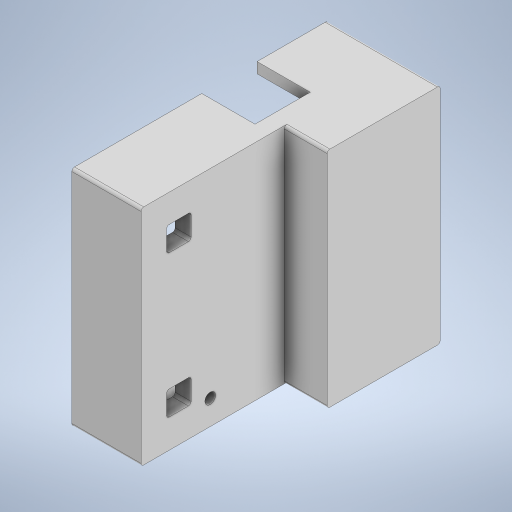
# Autodesk Inventor part: Part1
Saved by Autodesk Inventor 2023 (Build 270158030, 158C)
## iProperties
Created: 2023-07-27
Part Number: Part1
Material: Generic
Document SubType Name: Modeling
Designer: Tropaion
Density: 1 g/cm^3
Appearance: Default
Author: Tropaion
Autodesk Inventor part; units mm, degrees
ref_plane "YZ Plane" through (0, 0, 0) normal (1, 0, 0) x (0, 1, 0)
ref_plane "XZ Plane" through (0, 0, 0) normal (0, 1, 0) x (-1, 0, 0)
ref_plane "XY Plane" through (0, 0, 0) normal (0, 0, 1) x (1, 0, 0)
sketch "Sketch2" plane through (0, 0, 0) normal (1, 0, 0) x (0, 1, 0)
  line L0 (5.574, -18.3788) -> (-36.426, -18.3788)
  line L1 (-36.426, -18.3788) -> (-36.426, -39.5888)
  line L2 (-36.426, -39.5888) -> (5.574, -39.5888)
  line L3 (5.574, -39.5888) -> (5.574, -18.3788)
  point P0 (0, 0)
  dimension "d0" = 42
  dimension "d1" = 21.21
  constraints: 8 end point, 2 parallel, 1 horizontal, 1 perpendicular
  measures "d0" distance of L2.end L1.end
  measures "d1" distance of L1.end L0.end
extrude "Extrusion1" add sketch "Sketch2" along normal blind 3
sketch "Sketch4" plane through (0, 0, 0) normal (-1, 0, 0) x (0, 0, 1)
  line L0 (-18.3788, -36.426) -> (-39.5888, -36.426) projected
  line L1 (-39.5888, 5.574) -> (-18.3788, 5.574) projected
  line L2 (-18.3788, -36.426) -> (-21.3788, -36.426)
  line L3 (-21.3788, -36.426) -> (-21.3788, 5.574)
  line L4 (-21.3788, 5.574) -> (-18.3788, 5.574)
  line L5 (-18.3788, 5.574) -> (-18.3788, -36.426)
  point P0 (0, 0)
  point P1 (-18.3788, 5.574)
  dimension "d5" = 3
  constraints: 8 end point, 2 parallel, 1 horizontal, 1 perpendicular, 1 point on line
  measures "d5" distance of L3.end L4.end
extrude "Extrusion2" add sketch "Sketch4" along normal blind 8.09
sketch "Sketch5" plane through (3, -36.426, -18.3788) normal (0, 0, 1) x (1, 0, 0)
  line L0 (0, 0) -> (-11.09, 0) projected
  line L1 (-11.09, 42) -> (0, 42) projected
  line L2 (-11.09, 0) -> (-8.09, 0)
  line L3 (-8.09, 0) -> (-8.09, 42)
  line L4 (-8.09, 42) -> (-11.09, 42)
  line L5 (-11.09, 42) -> (-11.09, 0)
  point P0 (-3, 36.426)
  dimension "d8" = 3
  constraints: 8 end point, 2 parallel, 1 horizontal, 1 perpendicular, 1 point on line
  measures "d8" distance of L4.end L3.end
extrude "Extrusion3" add sketch "Sketch5" along normal blind 26.9
sketch "Sketch6" plane through (-8.09, 0, 0) normal (-1, 0, 0) x (0, 0, 1)
  line L0 (8.5212, 5.574) -> (8.5212, -36.426) projected
  line L1 (-21.3788, 5.574) -> (8.5212, 5.574)
  line L2 (8.5212, 5.574) -> (8.5212, 3.574)
  line L3 (8.5212, 3.574) -> (-21.3788, 3.574)
  line L4 (-21.3788, 3.574) -> (-21.3788, 5.574)
  point P0 (0, 0)
  dimension "d11" = 2
  constraints: 8 end point, 2 parallel, 1 horizontal, 1 perpendicular, 1 point on line
  measures "d11" distance of L1.end L2.end
extrude "Extrusion4" add sketch "Sketch6" along normal blind 10
sketch "Sketch7" plane through (0, 0, 0) normal (-1, 0, 0) x (0, 0, 1)
  line L0 (-21.3788, -36.426) -> (-21.3788, 5.574) projected
  line L1 (-39.5888, 5.574) -> (-21.3788, 5.574)
  line L2 (-21.3788, 5.574) -> (-21.3788, 3.574)
  line L3 (-21.3788, 3.574) -> (-39.5888, 3.574)
  line L4 (-39.5888, 3.574) -> (-39.5888, 5.574)
  point P0 (0, 0)
  dimension "d14" = 2
  constraints: 8 end point, 2 parallel, 1 horizontal, 1 perpendicular, 1 point on line
  measures "d14" distance of L1.end L2.end
extrude "Extrusion5" add sketch "Sketch7" along normal blind 18.09
sketch "Sketch8" plane through (-8.09, 0, 0) normal (-1, 0, 0) x (0, 0, 1)
  line L0 (-18.3788, -36.426) -> (8.5212, -36.426) projected
  line L1 (-21.3788, -36.426) -> (-21.3788, 3.574) projected
  line L2 (8.5212, -36.426) -> (-21.3788, -36.426)
  line L3 (-21.3788, -36.426) -> (-21.3788, -34.026)
  line L4 (-21.3788, -34.026) -> (8.5212, -34.026)
  line L5 (8.5212, -34.026) -> (8.5212, -36.426)
  point P0 (0, 0)
  dimension "d17" = 2.4
  constraints: 8 end point, 2 parallel, 1 horizontal, 1 perpendicular, 1 point on line
  measures "d17" distance of L2.end L3.end
extrude "Extrusion6" add sketch "Sketch8" along normal blind 10
sketch "Sketch9" plane through (0, 0, 0) normal (-1, 0, 0) x (0, 0, 1)
  line L0 (-39.5888, -36.426) -> (-39.5888, 5.574) projected
  line L1 (-21.3788, 3.574) -> (-21.3788, -34.026) projected
  line L2 (-39.5888, -36.426) -> (-21.3788, -36.426)
  line L3 (-21.3788, -36.426) -> (-21.3788, -34.026)
  line L4 (-21.3788, -34.026) -> (-39.5888, -34.026)
  line L5 (-39.5888, -34.026) -> (-39.5888, -36.426)
  point P0 (0, 0)
  constraints: 8 end point, 2 parallel, 1 horizontal, 1 perpendicular
extrude "Extrusion7" add sketch "Sketch9" along normal blind 18.09
sketch "Sketch10" plane through (-8.09, 0, 0) normal (-1, 0, 0) x (0, 0, 1)
  line L0 (-39.5888, 3.574) -> (8.5212, 3.574) projected
  line L1 (8.5212, -34.026) -> (-39.5888, -34.026) projected
  line L2 (8.5212, 3.574) -> (6.1212, 3.574)
  line L3 (6.1212, 3.574) -> (6.1212, -34.026)
  line L4 (6.1212, -34.026) -> (8.5212, -34.026)
  line L5 (8.5212, -34.026) -> (8.5212, 3.574)
  point P0 (0, 0)
  dimension "d22" = 2.4
  constraints: 8 end point, 2 parallel, 1 horizontal, 1 perpendicular, 1 point on line
  measures "d22" distance of L4.end L3.end
extrude "Extrusion8" add sketch "Sketch10" along normal blind 10
sketch "Sketch11" plane through (0, 0, 0) normal (-1, 0, 0) x (0, 0, 1)
  line L0 (-39.5888, 3.574) -> (6.1212, 3.574) projected
  line L1 (6.1212, -34.026) -> (-39.5888, -34.026) projected
  line L2 (-39.5888, 3.574) -> (-37.1888, 3.574)
  line L3 (-37.1888, 3.574) -> (-37.1888, -34.026)
  line L4 (-37.1888, -34.026) -> (-39.5888, -34.026)
  line L5 (-39.5888, -34.026) -> (-39.5888, 3.574)
  point P0 (0, 0)
  dimension "d25" = 2.4
  constraints: 8 end point, 2 parallel, 1 horizontal, 1 perpendicular, 1 point on line
  measures "d25" distance of L3.end L4.end
extrude "Extrusion9" add sketch "Sketch11" along normal blind 18.09
sketch "Sketch13" plane through (3, -36.426, -39.5888) normal (0, 0, -1) x (-1, 0, 0)
  line L0 (21.09, 40) -> (21.09, 2.4) projected
  line L1 (21.09, 3.2) -> (3.09, 3.2)
  line L2 (3.09, 3.2) -> (3.09, 16.4)
  line L3 (3.09, 16.4) -> (21.09, 16.4)
  line L4 (21.09, 16.4) -> (21.09, 3.2)
  line L5 (21.09, 0) -> (0, 0) projected
  point P0 (3, 36.426)
  dimension "d28" = 18
  dimension "d29" = 13.2
  dimension "d30" = 3.2
  constraints: 8 end point, 2 parallel, 1 horizontal, 1 perpendicular, 1 point on line
  measures "d28" distance of L2.end L3.end
  measures "d29" distance of L1.end L2.end
  measures "d30" distance between parallel lines of L5 L1
extrude "RJ12" cut sketch "Sketch13" against normal blind 2.4
sketch "Sketch14" plane through (3, -36.426, -39.5888) normal (0, 0, -1) x (-1, 0, 0)
  line L0 (21.09, 0) -> (21.09, 42) projected
  line L1 (21.09, 39.5) -> (5.89, 39.5)
  line L2 (5.89, 39.5) -> (5.89, 25.6)
  line L3 (5.89, 25.6) -> (21.09, 25.6)
  line L4 (21.09, 25.6) -> (21.09, 39.5)
  line L5 (21.09, 42) -> (0, 42) projected
  point P0 (3, 36.426)
  point P1 (21.09, 25.6)
  dimension "d33" = 15.2
  dimension "d34" = 13.9
  dimension "d35" = 2.5
  constraints: 8 end point, 2 parallel, 1 horizontal, 1 perpendicular, 1 point on line
  measures "d33" distance of L3.end L2.end
  measures "d34" distance of L2.end L1.end
  measures "d35" distance between parallel lines of L5 L1
extrude "PowerConnector" cut sketch "Sketch14" against normal blind 2.4
sketch "Sketch15" plane through (3, -36.426, -39.5888) normal (0, 0, -1) x (-1, 0, 0)
  line L0 (5.89, 39.5) -> (5.89, 25.6) projected
  line L1 (5.89, 33.6) -> (3.39, 33.6)
  line L2 (3.39, 33.6) -> (3.39, 31.6)
  line L3 (3.39, 31.6) -> (5.89, 31.6)
  line L4 (5.89, 31.6) -> (5.89, 33.6)
  line L5 (5.89, 39.5) -> (21.09, 39.5) projected
  point P0 (3, 36.426)
  point P1 (4.64, 33.6)
  dimension "d38" = 2.5
  dimension "d39" = 2
  dimension "d40" = 5.9
  constraints: 8 end point, 2 parallel, 1 horizontal, 1 midpoint, 1 perpendicular, 1 point on line
  measures "d38" distance of L3.end L2.end
  measures "d39" distance of L2.end L1.end
  measures "d40" distance from line of point (4.64, 33.6) L5
extrude "PowerConnector2" cut sketch "Sketch15" against normal blind 2.4
sketch "Sketch16" plane through (3, 5.574, -18.3788) normal (0, 1, 0) x (1, 0, 0)
  line L0 (-21.09, 18.81) -> (-21.09, -24.5) projected
  line L1 (-21.09, 7.91) -> (-11.09, 7.91)
  line L2 (-11.09, 7.91) -> (-11.09, -2.49)
  line L3 (-11.09, -2.49) -> (-21.09, -2.49)
  line L4 (-21.09, -2.49) -> (-21.09, 7.91)
  line L5 (-21.09, 21.21) -> (0, 21.21) projected
  point P0 (-3, -18.3788)
  dimension "d43" = 10
  dimension "d44" = 10.4
  dimension "d45" = 13.3
  constraints: 8 end point, 2 parallel, 1 horizontal, 1 perpendicular, 1 point on line
  measures "d43" distance of L2.end L3.end
  measures "d44" distance of L1.end L2.end
  measures "d45" distance between parallel lines of L5 L1
extrude "USBC" cut sketch "Sketch16" against normal blind 2.4
sketch "Sketch17" plane through (-5.09, -36.426, -18.3788) normal (1, 0, 0) x (0, 0, -1)
  line L0 (-17.5, 36.75) -> (-22.1, 36.75)
  line L1 (-22.1, 36.75) -> (-22.1, 32.15)
  line L2 (-22.1, 32.15) -> (-17.5, 32.15)
  line L3 (-17.5, 32.15) -> (-17.5, 36.75)
  line L4 (0, 42) -> (-26.9, 42) projected
  line L5 (-26.9, 0) -> (-26.9, 42) projected
  point P0 (-18.3788, 36.426)
  dimension "d48" = 4.6
  dimension "d49" = 4.6
  dimension "d50" = 5.25
  dimension "d51" = 4.8
  constraints: 8 end point, 2 parallel, 1 horizontal, 1 perpendicular
  measures "d48" distance of L2.end L1.end
  measures "d49" distance of L1.end L0.end
  measures "d50" distance between parallel lines of L4 L0
  measures "d51" distance between parallel lines of L5 L1
extrude "ResetButton" cut sketch "Sketch17" against normal blind 6.4
sketch "Sketch19" plane through (-5.09, -36.426, -18.3788) normal (1, 0, 0) x (0, 0, -1)
  line L0 (-17.5, 10) -> (-22.1, 10)
  line L1 (-22.1, 10) -> (-22.1, 5.4)
  line L2 (-22.1, 5.4) -> (-17.5, 5.4)
  line L3 (-17.5, 5.4) -> (-17.5, 10)
  line L4 (-26.9, 0) -> (-26.9, 42) projected
  line L5 (0, 0) -> (-26.9, 0) projected
  point P0 (-18.3788, 36.426)
  dimension "d54" = 4.6
  dimension "d55" = 4.6
  dimension "d56" = 4.8
  dimension "d57" = 5.4
  constraints: 8 end point, 2 parallel, 1 horizontal, 1 perpendicular
  measures "d54" distance of L2.end L1.end
  measures "d55" distance of L1.end L0.end
  measures "d56" distance between parallel lines of L4 L1
  measures "d57" distance between parallel lines of L2 L5
extrude "ZigbeeButton" cut sketch "Sketch19" against normal blind 6.4
fillet "Fillet1" radius 0.5 8 edges at (-6.59, -31.026, 3.7212) (-6.59, -4.276, 3.7212) (-6.59, 0.324, 3.7212) (-6.59, -26.426, 3.7212) (-6.59, -31.026, -0.8788) (-6.59, -4.276, -0.8788) (-6.59, -26.426, -0.8788) (-6.59, 0.324, -0.8788)
fillet "Fillet2" radius 0.5 2 edges at (-11.59, 5.574, 8.5212) (-11.59, -36.426, 8.5212)
fillet "Fillet3" radius 0.5 2 edges at (-7.545, 5.574, -39.5888) (-7.545, -36.426, -39.5888)
sketch "Sketch20" plane through (-5.09, -36.426, -18.3788) normal (1, 0, 0) x (0, 0, -1)
  circle A0 centre (-13.9, 4.6) radius 1
  line L0 (0, 0) -> (-26.4, 0) projected
  line L1 (-26.9, 0.5) -> (-26.9, 41.5) projected
  point P0 (-18.3788, 36.426)
  dimension "d63" = 2
  dimension "d64" = 4.6
  dimension "d65" = 13
  constraints: 1 centre point
  measures "d63" diameter of A0
  measures "d64" distance from line of L0 A0.centre
  measures "d65" distance from line of L1 A0.centre
extrude "LED" cut sketch "Sketch20" against normal blind 6.4
sketch "Sketch21" plane through (-18.09, 3.574, 6.1212) normal (0, -1, 0) x (1, 0, 0)
  line L0 (1, -13.5) -> (2, -13.5)
  line L1 (2, -13.5) -> (2, -8.5)
  line L2 (2, -8.5) -> (1, -8.5)
  line L3 (1, -8.5) -> (1, -13.5)
  line L4 (0, -22.01) -> (0, 0) projected
  line L5 (10, 0) -> (0, 0) projected
  point P0 (18.09, -6.1212)
  point P1 (1, -11)
  dimension "d68" = 1
  dimension "d69" = 5
  dimension "d70" = 1
  dimension "d71" = 11
  constraints: 8 end point, 2 parallel, 1 horizontal, 1 midpoint, 1 perpendicular
  measures "d68" distance of L2.end L1.end
  measures "d69" distance of L1.end L0.end
  measures "d70" distance from line of L4 point (1, -11)
  measures "d71" distance from line of L5 point (1, -11)
extrude "Extrusion17" cut sketch "Sketch21" against normal blind 0.5
sketch "Sketch22" plane through (-8.09, -34.026, -21.3788) normal (0, 1, 0) x (1, 0, 0)
  line L0 (-9, -19) -> (-8, -19)
  line L1 (-8, -19) -> (-8, -14)
  line L2 (-8, -14) -> (-9, -14)
  line L3 (-9, -14) -> (-9, -19)
  line L4 (-10, -27.5) -> (-10, 15.81) projected
  line L5 (-10, -27.5) -> (0, -27.5) projected
  point P0 (8.09, -21.3788)
  point P1 (-9, -16.5)
  dimension "d74" = 1
  dimension "d75" = 5
  dimension "d76" = 1
  dimension "d77" = 11
  constraints: 8 end point, 2 parallel, 1 horizontal, 1 midpoint, 1 perpendicular
  measures "d74" distance of L2.end L1.end
  measures "d75" distance of L1.end L0.end
  measures "d76" distance between parallel lines of L4 L3
  measures "d77" distance from line of L5 point (-9, -16.5)
extrude "Extrusion18" cut sketch "Sketch22" against normal blind 0.5
sketch "Sketch23" plane through (-8.09, -34.026, -21.3788) normal (0, 1, 0) x (1, 0, 0)
  line L0 (-9, 7.81) -> (-8, 7.81)
  line L1 (-8, 7.81) -> (-8, 12.81)
  line L2 (-8, 12.81) -> (-9, 12.81)
  line L3 (-9, 12.81) -> (-9, 7.81)
  line L4 (-10, -27.5) -> (-10, 15.81) projected
  line L5 (8.09, 15.81) -> (-10, 15.81) projected
  point P0 (8.09, -21.3788)
  point P1 (-9, 10.31)
  dimension "d80" = 1
  dimension "d81" = 5
  dimension "d82" = 1
  dimension "d83" = 5.5
  constraints: 8 end point, 2 parallel, 1 horizontal, 1 midpoint, 1 perpendicular
  measures "d80" distance of L2.end L1.end
  measures "d81" distance of L1.end L0.end
  measures "d82" distance between parallel lines of L4 L3
  measures "d83" distance from line of point (-9, 10.31) L5
extrude "Extrusion19" cut sketch "Sketch23" against normal blind 0.5
sketch "Sketch24" plane through (-8.09, 3.574, -21.3788) normal (0, -1, 0) x (1, 0, 0)
  line L0 (-9, -12.81) -> (-8, -12.81)
  line L1 (-8, -12.81) -> (-8, -7.81)
  line L2 (-8, -7.81) -> (-9, -7.81)
  line L3 (-9, -7.81) -> (-9, -12.81)
  line L4 (-10, -15.81) -> (-10, -4.91) projected
  line L5 (-10, -15.81) -> (8.09, -15.81) projected
  point P0 (8.09, 21.3788)
  point P1 (-10, -10.36)
  point P2 (-9, -10.31)
  dimension "d86" = 1
  dimension "d87" = 5
  dimension "d88" = 1
  dimension "d89" = 5.5
  constraints: 8 end point, 2 midpoint, 2 parallel, 1 horizontal, 1 perpendicular
  measures "d86" distance of L2.end L1.end
  measures "d87" distance of L1.end L0.end
  measures "d88" distance from line of point (-10, -10.36) L3
  measures "d89" distance from line of L5 point (-9, -10.31)
extrude "Extrusion20" cut sketch "Sketch24" against normal blind 0.5
fillet "Fillet4" radius 0.5 2 edges at (-1.045, 5.574, -18.3788) (-1.045, -36.426, -18.3788)
body "Solid1"
